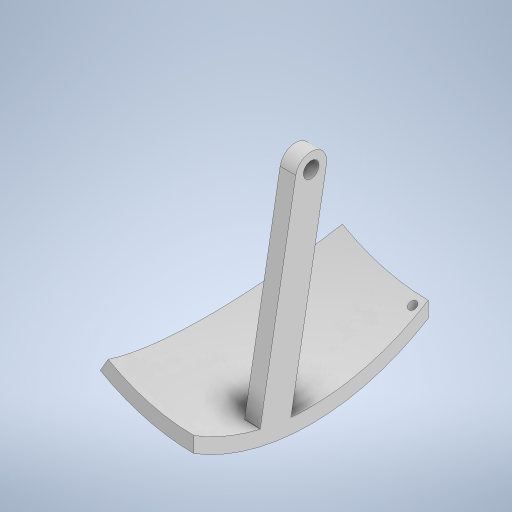
# Autodesk Inventor part: 受動歩行_ver4
Saved by Autodesk Inventor 2023 (Build 270158000, 158)
## iProperties
Created: 2024-06-12
Part Number: 受動歩行_ver4
Material: 一般
Document SubType Name: Modeling
Designer: babar
Density: 1 g/cm^3
Appearance: 既定
Author: babar
Autodesk Inventor part; units mm, degrees
ref_plane "YZ Plane" through (0, 0, 0) normal (1, 0, 0) x (0, 1, 0)
ref_plane "XZ Plane" through (0, 0, 0) normal (0, 1, 0) x (-1, 0, 0)
ref_plane "XY Plane" through (0, 0, 0) normal (0, 0, 1) x (1, 0, 0)
sketch "スケッチ1" plane through (0, 0, 0) normal (1, 0, 0) x (0, 1, 0)
  line L0 (-110, 0) -> (-125, 0)
  line L1 (-110, 75) -> (-120, 75)
  arc A0 (-120, 75) -> (-120, -75) centre (2.1096, 0) ccw
  line L2 (0, 75) -> (0, -75)
  line L3 (-110, -75) -> (-120, -75)
  arc A1 (-110, 75) -> (-110, -75) centre (10, 0) ccw
  point P0 (0, 0)
  point P1 (0, 0)
  dimension "d0" = 150
  dimension "d2" = 0
  dimension "d4" = 10
  dimension "d35" = 20
  constraints: 8 end point, 4 point on circle, 3 horizontal, 2 centre point, 1 coincident, 1 midpoint, 1 vertical
  measures "d0" distance of L1.start L3.start
  measures "d2" vertical distance of point (0, 0) L0.start
  measures "d4" distance of L1.start L1.end
  measures "d35" diameter of point (10, 0) point (0, 0)
revolve "回転1" add sketch "スケッチ1" angle 30 about axis through (0, 0, 75) along (0, 0, -1)
sketch "スケッチ2" plane through (0, -120, -75) normal (1, 0, 0) x (0, 0, -1)
  line L0 (-75, 120) -> (-97.7479, -9.0098) construction
  line L1 (-84.8481, 121.7365) -> (-107.596, -7.2733)
  line L2 (-87.8998, -10.7463) -> (-65.1519, 118.2635)
  arc A0 (-65.1519, 118.2635) -> (-84.8481, 121.7365) centre (-75, 120) ccw
  arc A1 (-107.596, -7.2733) -> (-87.8998, -10.7463) centre (-97.7479, -9.0098) ccw
  line L3 (-75, 120) -> (56, 120) construction
  point P0 (-86.374, 55.4951)
  dimension "d6" = 131
  dimension "d7" = 100
  dimension "d8" = 20
  constraints: 10 end point, 4 point on circle, 4 tangent, 2 centre point, 1 equal length, 1 horizontal, 1 midpoint, 1 parallel
  measures "d6" distance of L0.start L0.end
  measures "d7" angle of L0 L3
  measures "d8" diameter of A1
extrude "押し出し1" add sketch "スケッチ2" against normal blind 10
sketch "スケッチ3" plane through (0, -120, 75) normal (1, 0, 0) x (0, 0, -1)
  point P0 (75, 120)
  point P1 (75, 120)
  constraints: 1 coincident
hole "穴1" at (0, 0, 0) direction (-1, 0, 0) diameter 10 end through all
sketch "スケッチ5" plane through (1.0548, 1.8269, 0) normal (-0.8660254, 0.5, 0) x (-0.5, -0.8660254, 0)
  ellipse E0 centre (7.1096, 0) end of major axis (7.1096, -5) minor radius 4.3301 projected
  line L0 (7.1096, 0) -> (186.6716, 22.6929)
  arc A0 (122.1096, -75) -> (122.1096, 75) centre (0, 0) ccw projected
  point P0 (2.1096, 0)
  point P1 (138, 16.5418)
  dimension "d27" = 138
  constraints: 2 end point, 1 point on line, 1 other
  measures "d27" horizontal distance of A0.centre point (138, 16.542)
hole "穴3" at (-67.9452, -117.6846, 16.5418) direction (0.8660254, -0.5, 0) diameter 4.8 depth 10
sketch "スケッチ6" plane through (0, 0, 0) normal (0, 1, 0) x (-1, 0, 0)
  line L0 (0, -75) -> (0, 12.9316) projected
  line L1 (0, -75) -> (55, -75) projected
  point P0 (0, 0)
  point P1 (5, -70)
  dimension "d36" = 5
  dimension "d37" = 5
  measures "d36" distance from line of L0 point (5, -70)
  measures "d37" distance from line of L1 point (5, -70)
hole "穴4" at (-5, 0, -70) direction (0, -1, 0) diameter 4.8 end through all
